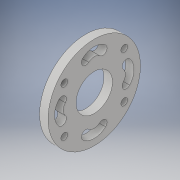
# Autodesk Inventor part: ballast_tutup
Saved by Autodesk Inventor 2019 (Build 230136000, 136)
## iProperties
Created: 2020-07-18
Part Number: ballast_tutup
Material: Generic
Document SubType Name: Modeling
Designer: Agus Prayudi
Density: 1 g/cm^3
Appearance: Default
Author: Agus Prayudi
Autodesk Inventor part; units mm, degrees
ref_plane "YZ Plane" through (0, 0, 0) normal (1, 0, 0) x (0, 1, 0)
ref_plane "XZ Plane" through (0, 0, 0) normal (0, 1, 0) x (-1, 0, 0)
ref_plane "XY Plane" through (0, 0, 0) normal (0, 0, 1) x (1, 0, 0)
sketch "Sketch2" plane through (0, 0, 0) normal (1, 0, 0) x (0, 1, 0)
  circle A0 centre (0, 0) radius 54.5
  circle A1 centre (-27.25, -35.3988) radius 3.5
  circle A2 centre (-27.25, 35.3988) radius 3.5
  circle A3 centre (27.25, -35.3988) radius 3.5
  circle A4 centre (27.25, 35.3988) radius 3.5
  circle A5 centre (0, 0) radius 21.5
  constraints: 6 centre point, 2 coincident
extrude "Extrusion4" add sketch "Sketch2" along normal blind 10
sketch "Sketch4" plane through (10, 0, 0) normal (1, 0, 0) x (0, 0, -1)
  circle A0 centre (0, 0) radius 54.5 projected
  circle A1 centre (0, 0) radius 21.5 projected
  arc A2 (10, 38) -> (-10, 38) centre (0, 26.8197) ccw construction
  arc A3 (13.4228, 41.8269) -> (-13.4228, 41.8269) centre (0, 26.8197) ccw
  arc A4 (6.5772, 34.1731) -> (-6.5772, 34.1731) centre (0, 26.8197) ccw
  arc A5 (6.5772, 34.1731) -> (13.4228, 41.8269) centre (10, 38) ccw
  arc A6 (-13.4228, 41.8269) -> (-6.5772, 34.1731) centre (-10, 38) ccw
  dimension "d28" = 15
  constraints: 10 point on circle, 5 centre point, 4 tangent
  measures "d28" radius of A2
extrude "Extrusion5" cut sketch "Sketch4" against normal blind 10 contours A5 A4 A6 A3
pattern_circular "Circular Pattern2" count 4 over 360 about axis through (0, 0, 0) along (1, 0, 0) of "Extrusion5"
sketch "Sketch5" plane through (10, 0, 0) normal (1, 0, 0) x (0, 0, -1)
  arc A0 (41.8269, 13.4228) -> (34.1731, 6.5772) centre (38, 10) ccw projected
  arc A1 (41.8269, -13.4228) -> (41.8269, 13.4228) centre (26.8197, 0) ccw projected
  arc A2 (34.1731, -6.5772) -> (41.8269, -13.4228) centre (38, -10) ccw projected
  arc A3 (34.1731, -6.5772) -> (34.1731, 6.5772) centre (26.8197, 0) ccw projected
  arc A4 (13.4228, -41.8269) -> (6.5772, -34.1731) centre (10, -38) ccw projected
  arc A5 (-13.4228, -41.8269) -> (13.4228, -41.8269) centre (0, -26.8197) ccw projected
  arc A6 (-6.5772, -34.1731) -> (-13.4228, -41.8269) centre (-10, -38) ccw projected
  arc A7 (-6.5772, -34.1731) -> (6.5772, -34.1731) centre (0, -26.8197) ccw projected
  arc A8 (-41.8269, -13.4228) -> (-34.1731, -6.5772) centre (-38, -10) ccw projected
  arc A9 (-41.8269, 13.4228) -> (-41.8269, -13.4228) centre (-26.8197, 0) ccw projected
  arc A10 (-34.1731, 6.5772) -> (-41.8269, 13.4228) centre (-38, 10) ccw projected
  arc A11 (-34.1731, 6.5772) -> (-34.1731, -6.5772) centre (-26.8197, 0) ccw projected
  arc A12 (-13.4228, 41.8269) -> (-6.5772, 34.1731) centre (-10, 38) ccw projected
  arc A13 (13.4228, 41.8269) -> (-13.4228, 41.8269) centre (0, 26.8197) ccw projected
  arc A14 (6.5772, 34.1731) -> (13.4228, 41.8269) centre (10, 38) ccw projected
  arc A15 (6.5772, 34.1731) -> (-6.5772, 34.1731) centre (0, 26.8197) ccw projected
  circle A16 centre (0, 0) radius 21.5 projected
  circle A17 centre (35.3988, 27.25) radius 3.5 projected
  circle A18 centre (-35.3988, 27.25) radius 3.5 projected
  circle A19 centre (-35.3988, -27.25) radius 3.5 projected
  circle A20 centre (35.3988, -27.25) radius 3.5 projected
  circle A21 centre (0, 0) radius 54.5 projected
sketch "Sketch6" plane through (10, 0, 0) normal (1, 0, 0) x (0, 0, -1)
  circle A0 centre (-35.3988, 27.25) radius 3.5 projected
  circle A1 centre (35.3988, 27.25) radius 3.5 projected
  circle A2 centre (-35.3988, -27.25) radius 3.5 projected
  circle A3 centre (35.3988, -27.25) radius 3.5 projected
  circle A4 centre (-35.3988, 27.25) radius 4
  circle A5 centre (35.3988, 27.25) radius 4
  circle A6 centre (-35.3988, -27.25) radius 4
  circle A7 centre (35.3988, -27.25) radius 4
  point P0 (0, 0)
  constraints: 4 centre point, 4 coincident
extrude "Extrusion6" cut sketch "Sketch6" against normal blind 10
body "Solid3"
